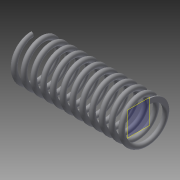
# Autodesk Inventor part: 3 in spring
Saved by Autodesk Inventor 2014 SP1 (Build 180222100, 222)
## iProperties
Created: 2014-01-31
Part Number: 3 in spring
Material: Generic
Document SubType Name: Modeling
Designer: Owner
Density: 1 g/cm^3
Appearance: Default
Author: Owner
Autodesk Inventor part; units mm, degrees
ref_plane "YZ Plane" through (0, 0, 0) normal (1, 0, 0) x (0, 1, 0)
ref_plane "XZ Plane" through (0, 0, 0) normal (0, 1, 0) x (-1, 0, 0)
ref_plane "XY Plane" through (0, 0, 0) normal (0, 0, 1) x (1, 0, 0)
sketch "Sketch1" plane through (0, 0, 0) normal (0, 0, 1) x (1, 0, 0)
  line L0 (0, 0) -> (30.6807, 0)
  line L1 (0, 0) -> (0, 12.7) construction
  circle A0 centre (0, 12.7) radius 1.5875
  dimension "d0" = 12.7
  dimension "d1" = 3.175
  constraints: 4 end point, 1 centre point, 1 coincident, 1 horizontal, 1 perpendicular
  measures "d0" distance of L0.start L1.end
  measures "d1" diameter of A0
coil "Coil1" sketch "Sketch1" operation add axis through (0, 0, 0) along (1, 0, 0) pitch 6.35 turns 12 hand right
sketch "Sketch2" plane through (0, 0, 0) normal (1, 0, 0) x (0, 1, 0)
  line L0 (-21.4545, 20.1834) -> (20.8964, 20.1834)
  line L1 (20.8964, 20.1834) -> (20.8964, -18.8192)
  line L2 (20.8964, -18.8192) -> (-21.4545, -18.8192)
  line L3 (-21.4545, -18.8192) -> (-21.4545, 20.1834)
  point P0 (0, 0)
  constraints: 8 end point, 2 parallel, 1 horizontal, 1 perpendicular
extrude "Extrusion1" cut sketch "Sketch2" against normal blind 25.4
ref_plane "Work Plane1" through (76.2, 0, 0) normal (-1, 0, 0) x (0, 0, 1)
sketch "Sketch3" plane through (76.2, 0, 0) normal (-1, 0, 0) x (0, 0, 1)
  line L0 (-21.6352, 24.3664) -> (43.9131, 24.3664)
  line L1 (43.9131, 24.3664) -> (43.9131, -35.6125)
  line L2 (43.9131, -35.6125) -> (-21.6352, -35.6125)
  line L3 (-21.6352, -35.6125) -> (-21.6352, 24.3664)
  point P0 (0, 0)
  constraints: 8 end point, 2 parallel, 1 horizontal, 1 perpendicular
extrude "Extrusion2" cut sketch "Sketch3" against normal blind 25.4
body "Solid1"
